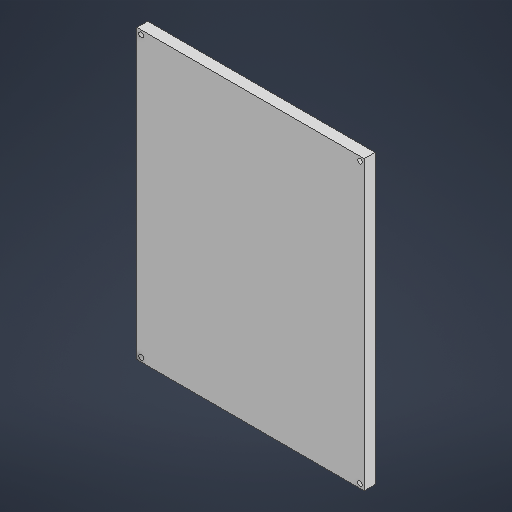
# Autodesk Inventor part: tapa
Saved by Autodesk Inventor 2026.3 (Build 303398000, 398)
## iProperties
Created: 2026-05-13
Part Number: tapa
Material: Genérico
Document SubType Name: Modeling
Designer: Santiago A
Density: 1 g/cm^3
Appearance: Valor por defecto
Author: Santiago A
Autodesk Inventor part; units mm, degrees
ref_plane "YZ Plane" through (0, 0, 0) normal (1, 0, 0) x (0, 1, 0)
ref_plane "XZ Plane" through (0, 0, 0) normal (0, 1, 0) x (-1, 0, 0)
ref_plane "XY Plane" through (0, 0, 0) normal (0, 0, 1) x (1, 0, 0)
sketch "Boceto3" plane through (0, 0, 0) normal (0, 0, 1) x (1, 0, 0)
  line L0 (0, 0) -> (94, 0)
  line L1 (94, 0) -> (94, -119)
  line L2 (94, -119) -> (0, -119)
  line L3 (0, -119) -> (0, 0)
  dimension "d18" = 94
  dimension "d19" = 119
  constraints: 8 end point, 2 parallel, 1 horizontal, 1 perpendicular
  measures "d18" distance of L1.end L2.end
  measures "d19" distance of L0.end L1.end
extrude "Extrusión3" add sketch "Boceto3" along normal blind 4.5
sketch "Boceto4" plane through (0, 0, 4.5) normal (0, 0, 1) x (1, 0, 0)
  line L0 (0, 0) -> (1.75, 0)
  line L1 (94, 0) -> (0, 0) projected
  line L2 (0, 0) -> (0, -1.75)
  line L3 (0, 0) -> (0, -119) projected
  line L4 (94, 0) -> (92.25, 0)
  line L5 (94, 0) -> (94, -1.75)
  line L6 (0, -119) -> (94, -119) projected
  line L7 (94, -119) -> (94, -117.25)
  line L8 (94, -119) -> (94, 0) projected
  line L9 (94, -119) -> (92.25, -119)
  circle A0 centre (92.25, -117.25) radius 1
  line L10 (0, -119) -> (1.75, -119)
  line L11 (0, -119) -> (0, -117.25)
  circle A1 centre (1.75, -117.25) radius 1
  circle A2 centre (1.75, -1.75) radius 1
  circle A3 centre (92.25, -1.75) radius 1
  dimension "d22" = 1.75
  dimension "d23" = 1.75
  dimension "d24" = 1.75
  dimension "d25" = 1.75
  dimension "d26" = 1.75
  dimension "d27" = 1.75
  dimension "d28" = 2
  dimension "d29" = 1.75
  dimension "d30" = 1.75
  dimension "d31" = 2
  dimension "d32" = 2
  dimension "d33" = 2
  constraints: 16 end point, 7 point on line, 4 centre point, 1 perpendicular
  measures "d22" distance of L0.start L0.end
  measures "d23" distance of L0.start L2.end
  measures "d24" distance of L1.start L4.end
  measures "d25" distance of L1.start L5.end
  measures "d26" distance of L6.end L7.end
  measures "d27" distance of L6.end L9.end
  measures "d28" diameter of A0
  measures "d29" distance of L3.end L10.end
  measures "d30" distance of L3.end L11.end
  measures "d31" diameter of A1
  measures "d32" diameter of A2
  measures "d33" diameter of A3
extrude "Extrusión4" cut sketch "Boceto4" against normal blind 8 contours A0 | A1 | A2 | A3
